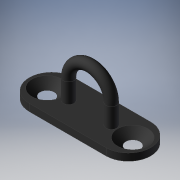
# Autodesk Inventor part: TKCb
Saved by Autodesk Inventor 2019 (Build 230136000, 136)
## iProperties
Created: 2024-03-12
Part Number: TKCb
Material: Generic
Catalog Web Link: www.cadenas.de
Description: TKCb-Mounting Brackets
Vendor: MISUMI
Document SubType Name: Modeling
Designer: psAdmin
Manufacturer: MISUMI
Mass: 0.865911 g
Surface Area: 11.9426 cm^2
Volume: 0.865911 cm^3
Density: 1 g/cm^3
Appearance: PSOLRGB-175-175-175
Category: PARTsolutions
Company: MISUMI
Title: TKCb
Author: Cadenas PARTsolutions
Comments: Mounting Brackets
PSOL_IDENT_0: {$CADENAS_DATA/23d-libs/misumi/metric/28_keys_magnets/tkc.prj},146 {VTYP=3D},{NB=TKCb},{LINA=TKCb},{
PSOL_IDENT_1: NN=TKCb},{DATE=30.03.2023 02:29:30},{GEOMDATE=15.03.2023 02:51:42},{VERSION=},{LINEID=10},{WBVAR=},{
PSOL_IDENT_2: WBNUMERIC=}  {NB=TKCb},{LINA=TKCb},{KT=DUMMY},{PN=TKCb},{TP=TKCb},{MAT=304 Stainless Steel},{MATAC=3
PSOL_IDENT_3: 04 Stainless Steel},{AC=M4-5 Flat Head Screw 2 pcs.},{RWL=20}
NB: TKCb
NN: TKCb
NT: Mounting Brackets
NBSYN: $PN.
LINA: TKCb
CATALOG: Misumi
PN: TKCb
TP: TKCb
MAT: 304 Stainless Steel
MATAC: 304 Stainless Steel
AC: M4-5 Flat Head Screw 2 pcs.
RWL: 20
SUPPLIER: MISUMI
ARTICLENO: TKCb
BOMINFO: TKCb
CREATOR: CADENAS GmbH
Autodesk Inventor part; units mm, degrees
sketch "Sketch_1" plane through (0, 0, 0) normal (0, 1, 0) x (-1, 0, 0)
  arc A0 (10.75, -6.25) -> (10.75, 6.25) centre (10.75, 0) ccw
  line L0 (10.75, 6.25) -> (-10.75, 6.25)
  arc A1 (-10.75, 6.25) -> (-10.75, -6.25) centre (-10.75, 0) ccw
  line L1 (-10.75, -6.25) -> (10.75, -6.25)
  constraints: 4 end point, 4 point on circle, 2 centre point
extrude "Extrusion1" add sketch "Sketch_1" along normal blind 2
sketch "Sketch_2" plane through (0, 2, 0) normal (0, 1, 0) x (1, 0, 0)
  circle A0 centre (-6, 0) radius 1.5
  constraints: 1 centre point
extrude "Extrusion2" add sketch "Sketch_2" along normal blind 5.5
sketch "Sketch_3" plane through (0, 2, 0) normal (0, 1, 0) x (1, 0, 0)
  circle A0 centre (6, 0) radius 1.5
  constraints: 1 centre point
extrude "Extrusion3" add sketch "Sketch_3" along normal blind 5.5
sketch "Sketch_4" plane through (0, 7.5, 0) normal (0, 1, 0) x (1, 0, 0)
  line L0 (0, 5) -> (0, -5)
  circle A0 centre (-6, 0) radius 1.5
  constraints: 2 end point, 1 centre point
revolve "Revolution1" add sketch "Sketch_4" angle 180 about axis through (0, 7.5, -5) along (0, 0, -1)
sketch "Sketch_5" plane through (0, 0, 0) normal (0, 0, 1) x (1, 0, 0)
  line L0 (-12, 0) -> (-12, 2)
  line L1 (-12, 2) -> (-7.75, 2)
  line L2 (-7.75, 2) -> (-10, 0)
  line L3 (-10, 0) -> (-12, 0)
  line L4 (-12, 0) -> (-12, 2)
  constraints: 10 end point
revolve "Revolution2" cut sketch "Sketch_5" angle 360 about axis through (-12, 0, 0) along (0, -1, 0)
sketch "Sketch_7" plane through (0, 0, 0) normal (0, 0, 1) x (1, 0, 0)
  line L0 (12, 0) -> (12, 2)
  line L1 (12, 2) -> (16.25, 2)
  line L2 (16.25, 2) -> (14, 0)
  line L3 (14, 0) -> (12, 0)
  line L4 (12, 0) -> (12, 2)
  constraints: 10 end point
revolve "Revolution3" cut sketch "Sketch_7" angle 360 about axis through (12, 0, 0) along (0, -1, 0)
ref_plane "cp1_XY" through (-12, 0, 0) normal (0, 1, 0) x (1, 0, 0)
ref_plane "cp1_YZ" through (-12, 0, 0) normal (1, 0, 0) x (0, 0, -1)
ref_plane "cp1_ZX" through (-12, 0, 0) normal (0, 0, -1) x (0, 1, 0)
ref_plane "cp2_XY" through (12, 0, 0) normal (0, 1, 0) x (1, 0, 0)
ref_plane "cp2_YZ" through (12, 0, 0) normal (1, 0, 0) x (0, 0, -1)
ref_plane "cp2_ZX" through (12, 0, 0) normal (0, 0, -1) x (0, 1, 0)
ref_plane "to_wire_XY" through (0, 13.5, 0) normal (1, 0, 0) x (0, 0, -1)
ref_plane "to_wire_YZ" through (0, 13.5, 0) normal (0, 0, -1) x (0, 1, 0)
ref_plane "to_wire_ZX" through (0, 13.5, 0) normal (0, 1, 0) x (1, 0, 0)
body "Solid1"
